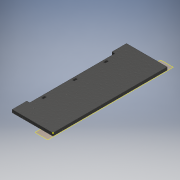
# Autodesk Inventor part: fronts-02
Saved by Autodesk Inventor 2018 (Build 220112000, 112)
## iProperties
Created: 2017-10-09
Part Number: fronts-02
Material: Generic
Document SubType Name: Modeling
Designer: HP
Density: 1 g/cm^3
Appearance: Fine Textured - Black
Author: HP
Autodesk Inventor part; units mm, degrees
ref_plane "YZ Plane" through (0, 0, 0) normal (1, 0, 0) x (0, 1, 0)
ref_plane "XZ Plane" through (0, 0, 0) normal (0, 1, 0) x (-1, 0, 0)
ref_plane "XY Plane" through (0, 0, 0) normal (0, 0, 1) x (1, 0, 0)
ref_plane "Work Plane1" through (0, 0, -5.5) normal (0, 0, 1) x (1, 0, 0)
sketch "Sketch1" plane through (0, 0, -5.5) normal (0, 0, 1) x (1, 0, 0)
  line L0 (0, 197) -> (0, 0) construction
  line L1 (0, 197) -> (-20, 197) construction
  line L2 (-20, 0) -> (-20, 197) construction
  line L3 (0, 0) -> (-20, 0) construction
  line L4 (0, 0) -> (-70, 0) construction
  line L5 (-70, 0) -> (-70, -5) construction
  line L6 (0, -5) -> (-70, -5) construction
  line L7 (0, 0) -> (0, -5) construction
  line L8 (-70, 197) -> (0, 197) construction
  line L9 (0, 197) -> (0, 202) construction
  line L10 (-70, 202) -> (0, 202) construction
  line L11 (-70, 197) -> (-70, 202) construction
  line L12 (0, 0) -> (0, 197)
  line L13 (0, 0) -> (-70, 0)
  line L14 (-70, 0) -> (-70, 25)
  line L15 (-70, 25) -> (-65, 25)
  line L16 (-65, 25) -> (-65, 172)
  line L17 (-65, 172) -> (-70, 172)
  line L18 (-70, 172) -> (-70, 197)
  line L19 (-70, 197) -> (0, 197)
  line L20 (-65, 0) -> (-65, -5) construction
  dimension "d1" = 0
  dimension "d2" = 0
  dimension "d3" = 25
  dimension "d4" = 25
  constraints: 16 end point, 6 perpendicular, 4 collinear, 1 point on line, 1 vertical
  measures "d1" distance from line of L12.start L4
  measures "d2" distance from line of L12.end L8
  measures "d3" distance between parallel lines of L15 L13
  measures "d4" distance between parallel lines of L17 L19
extrude "Extrusion1" add sketch "Sketch1" along normal blind 5
sketch "Sketch2" plane through (0, 0, -0.5) normal (0, 0, 1) x (1, 0, 0)
  point P0 (0, 0)
sketch "Sketch3" plane through (0, 0, -5.5) normal (0, 0, -1) x (-1, 0, 0)
  line L0 (0, 0) -> (0, 197) construction
  line L1 (0, 0) -> (20, 0) construction
  line L2 (20, 197) -> (20, 0) construction
  line L3 (0, 197) -> (20, 197) construction
  line L4 (10, 197) -> (10, 0) construction
  line L5 (0, 0) -> (0, 197) construction
  line L6 (0, 98.5) -> (20, 98.5) construction
  point P0 (10, 98.5)
  point P1 (10, 177)
  point P2 (10, 20)
  dimension "d7" = 20
  dimension "d8" = 20
  constraints: 5 midpoint, 4 end point, 2 point on line
  measures "d7" distance from line of point (10, 177) L3
  measures "d8" distance from line of point (10, 20) L1
hole "Hole1" [suppressed]
sketch "Sketch4" plane through (-65, 25, -5.5) normal (-1, 0, 0) x (0, 0, 1)
  line L0 (0, 147) -> (0, 0) construction
  line L1 (0, 0) -> (5, 0) construction
  line L2 (5, 147) -> (5, 0) construction
  line L3 (0, 147) -> (5, 147) construction
  line L4 (2.5, 0) -> (2.5, 147) construction
  line L5 (5, 147) -> (5, 0) construction
  line L6 (5, 73.5) -> (0, 73.5) construction
  point P0 (5.5, -25)
  point P1 (2.5, 73.5)
  point P2 (2.5, 127)
  point P3 (2.5, 20)
  dimension "d16" = 20
  dimension "d17" = 20
  constraints: 5 midpoint, 4 end point, 2 point on line
  measures "d16" distance from line of point (2.5, 20) L1
  measures "d17" distance from line of point (2.5, 127) L3
hole "Hole2" at (-65, 98.5, -3) at (-65, 152, -3) at (-65, 45, -3) direction (1, 0, 0) diameter 2.459 depth 8.8 tip angle 118 thread size "M3x0.5" class "6H" standard "ISO Metric profile"
sketch "Sketch5" plane through (0, 0, -0.5) normal (0, 0, 1) x (1, 0, 0)
  line L0 (-56.2, 46.2295) -> (-65, 46.2295) construction
  line L1 (-56.2, 43.7705) -> (-65, 43.7705) construction
  line L2 (-56.2, 99.7295) -> (-65, 99.7295) construction
  line L3 (-56.2, 97.2705) -> (-65, 97.2705) construction
  line L4 (-56.2, 153.2295) -> (-65, 153.2295) construction
  line L5 (-56.2, 150.7705) -> (-65, 150.7705) construction
  line L6 (-65, 43.7705) -> (-65, 46.2295) construction
  line L7 (-65, 43.7705) -> (-65, 46.2295) construction
  line L8 (-65, 45) -> (-57.2589, 45) construction
  line L9 (-62, 42.15) -> (-59, 42.15)
  line L10 (-59, 42.15) -> (-59, 47.85)
  line L11 (-59, 47.85) -> (-62, 47.85)
  line L12 (-62, 47.85) -> (-62, 42.15)
  line L13 (-65, 150.7705) -> (-65, 153.2295) construction
  line L14 (-65, 150.7705) -> (-65, 153.2295) construction
  line L15 (-65, 152) -> (-56.2589, 152) construction
  line L16 (-62, 149.15) -> (-59, 149.15)
  line L17 (-59, 149.15) -> (-59, 154.85)
  line L18 (-59, 154.85) -> (-62, 154.85)
  line L19 (-62, 154.85) -> (-62, 149.15)
  line L20 (-65, 97.2705) -> (-65, 99.7295) construction
  line L21 (-65, 97.2705) -> (-65, 99.7295) construction
  line L22 (-65, 98.5) -> (-54.9007, 98.5) construction
  line L23 (-62, 95.65) -> (-59, 95.65)
  line L24 (-59, 95.65) -> (-59, 101.35)
  line L25 (-59, 101.35) -> (-62, 101.35)
  line L26 (-62, 101.35) -> (-62, 95.65)
  point P0 (0, 0)
  dimension "d25" = 5.7
  dimension "d26" = 3
  dimension "d27" = 3
  dimension "d28" = 5.7
  dimension "d29" = 3
  dimension "d30" = 3
  dimension "d31" = 5.7
  dimension "d32" = 3
  dimension "d33" = 3
  constraints: 40 end point, 9 equal length, 6 horizontal, 3 midpoint, 3 perpendicular, 3 other
  measures "d25" distance between parallel lines of L9 L11
  measures "d26" distance between parallel lines of L12 L6
  measures "d27" distance between parallel lines of L10 L12
  measures "d28" distance between parallel lines of L16 L18
  measures "d29" distance between parallel lines of L19 L13
  measures "d30" distance between parallel lines of L17 L19
  measures "d31" distance between parallel lines of L23 L25
  measures "d32" distance between parallel lines of L26 L20
  measures "d33" distance between parallel lines of L24 L26
extrude "Extrusion2" cut sketch "Sketch5" against normal through all
sketch "Sketch6" plane through (0, 0, -5.5) normal (0, 0, -1) x (-1, 0, 0)
  line L0 (35, 87) -> (0, 87) projected
  arc A0 (35, 87) -> (35, 95) centre (35, 91) ccw projected
  line L1 (0, 95) -> (35, 95) projected
  line L2 (0, 95) -> (0, 87)
  line L3 (0, 0) -> (0, 197) projected
  line L4 (65, 153) -> (65, 110) construction
  line L5 (70, 153) -> (65, 153) construction
  line L6 (70, 110) -> (70, 153) construction
  line L7 (70, 110) -> (65, 110) construction
  line L8 (70, 131.5) -> (0, 131.5) construction
  line L9 (62, 139) -> (47, 139)
  line L10 (47, 139) -> (47, 124)
  line L11 (47, 124) -> (62, 124)
  line L12 (62, 124) -> (62, 139)
  dimension "d36" = 15
  dimension "d37" = 15
  dimension "d38" = 3
  constraints: 12 end point, 2 parallel, 2 perpendicular, 1 collinear, 1 horizontal, 1 midpoint, 1 point on line, 1 other
  measures "d36" distance of L11.end L10.end
  measures "d37" distance of L10.end L9.end
  measures "d38" distance between parallel lines of L4 L12
extrude "Extrusion3" [suppressed]
equation "\"d4\" = d3"
equation "\"d5\" = plate_thickness"
equation "\"d8\" = d7"
equation "\"d17\" = d16"
equation "\"plate_thickness\" = 5"
equation "\"basic_plate_offset\" = 0"
equation "\"ABS_tolerance\" = 0"
equation "\"laser_cutter_thickness\" = 0.1"
body "Solid1"
